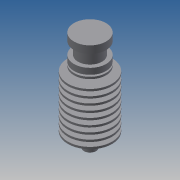
# Autodesk Inventor part: heat sink
Saved by Autodesk Inventor 2013 (Build 170138000, 138)
## iProperties
Created: 2017-04-01
Part Number: heat sink
Material: Generic
Document SubType Name: Modeling
Designer: employee
Density: 1 g/cm^3
Author: employee
Autodesk Inventor part; units mm, degrees
ref_plane "YZ Plane" through (0, 0, 0) normal (1, 0, 0) x (0, 1, 0)
ref_plane "XZ Plane" through (0, 0, 0) normal (0, 1, 0) x (-1, 0, 0)
ref_plane "XY Plane" through (0, 0, 0) normal (0, 0, 1) x (1, 0, 0)
sketch "Sketch1" plane through (0, 0, 0) normal (1, 0, 0) x (0, 1, 0)
  line L0 (0, -49.8) -> (0, 0)
  line L1 (0, 0) -> (-8, 0)
  line L2 (-8, 0) -> (-8, -3.7)
  line L3 (-8, -3.7) -> (-6, -3.7)
  line L4 (-6, -3.7) -> (-6, -9.7)
  line L5 (-6, -9.7) -> (-8, -9.7)
  line L6 (-8, -9.7) -> (-8, -12.7)
  line L7 (-8, -12.7) -> (-3, -12.7)
  line L8 (-3, -12.7) -> (-3, -49.8)
  line L9 (-3, -49.8) -> (0, -49.8)
  line L10 (-3, -42.7) -> (-11, -42.7)
  line L11 (-11, -42.7) -> (-11, -41.7)
  line L12 (-11, -41.7) -> (-3, -41.7)
  line L13 (-3, -41.7) -> (-3, -42.7)
  line L14 (-3, -39.575) -> (-11, -39.575)
  line L15 (-11, -39.575) -> (-11, -38.575)
  line L16 (-11, -38.575) -> (-3, -38.575)
  line L17 (-3, -38.575) -> (-3, -39.575)
  line L18 (-3, -27.075) -> (-11, -27.075)
  line L19 (-11, -27.075) -> (-11, -26.075)
  line L20 (-11, -26.075) -> (-3, -26.075)
  line L21 (-3, -26.075) -> (-3, -27.075)
  line L22 (-3, -20.825) -> (-11, -20.825)
  line L23 (-11, -20.825) -> (-11, -19.825)
  line L24 (-11, -19.825) -> (-3, -19.825)
  line L25 (-3, -19.825) -> (-3, -20.825)
  line L26 (-3, -30.2) -> (-11, -30.2)
  line L27 (-11, -30.2) -> (-11, -29.2)
  line L28 (-11, -29.2) -> (-3, -29.2)
  line L29 (-3, -29.2) -> (-3, -30.2)
  line L30 (-3, -33.325) -> (-11, -33.325)
  line L31 (-11, -33.325) -> (-11, -32.325)
  line L32 (-11, -32.325) -> (-3, -32.325)
  line L33 (-3, -32.325) -> (-3, -33.325)
  line L34 (-3, -36.45) -> (-11, -36.45)
  line L35 (-11, -36.45) -> (-11, -35.45)
  line L36 (-11, -35.45) -> (-3, -35.45)
  line L37 (-3, -35.45) -> (-3, -36.45)
  line L38 (-3, -23.95) -> (-11, -23.95)
  line L39 (-11, -23.95) -> (-11, -22.95)
  line L40 (-11, -22.95) -> (-3, -22.95)
  line L41 (-3, -22.95) -> (-3, -23.95)
  line L42 (-3, -17.7) -> (-11, -17.7)
  line L43 (-11, -17.7) -> (-11, -16.7)
  line L44 (-11, -16.7) -> (-3, -16.7)
  line L45 (-3, -16.7) -> (-3, -17.7)
  line L46 (-11, -17.7) -> (-11, -19.825) construction
  line L47 (-11, -20.825) -> (-11, -22.95) construction
  line L48 (-11, -23.95) -> (-11, -26.075) construction
  line L49 (-11, -27.075) -> (-11, -29.2) construction
  line L50 (-11, -30.2) -> (-11, -32.325) construction
  line L51 (-11, -33.325) -> (-11, -35.45) construction
  line L52 (-11, -36.45) -> (-11, -38.575) construction
  line L53 (-11, -41.7) -> (-11, -39.575) construction
  line L54 (-8, -13.575) -> (-3, -13.575)
  line L55 (-3, -13.575) -> (-3, -14.575)
  line L56 (-3, -14.575) -> (-8, -14.575)
  line L57 (-8, -14.575) -> (-8, -13.575)
  line L58 (-8, -14.575) -> (-8, -16.7) construction
  line L59 (-3, -42.7) -> (-2.05, -42.7)
  line L60 (-2.05, -42.7) -> (-2.05, -44.8)
  line L61 (-2.05, -44.8) -> (-3, -44.8)
  line L62 (-3, -44.8) -> (-3, -42.7)
  dimension "d0" = 3.7
  dimension "d2" = 6
  dimension "d3" = 3
  dimension "d4" = 8
  dimension "d5" = 6
  dimension "d6" = 3
  dimension "d7" = 49.8
  dimension "d9" = 1
  dimension "d11" = 26
  dimension "d12" = 7.1
  dimension "d13" = 11
  dimension "d14" = 5
  dimension "d15" = 2.05
  constraints: 124 end point, 30 parallel, 27 equal length, 12 perpendicular, 11 horizontal, 8 collinear, 2 vertical, 1 point on line, 13 other
  measures "d0" distance of L1.end L2.end
  measures "d2" distance of L3.end L4.end
  measures "d3" distance of L5.end L6.end
  measures "d4" distance of L0.end L1.end
  measures "d5" distance between parallel lines of L0 L4
  measures "d7" distance from line of L0.start L1
  measures "d9" distance of L10.end L11.end
  measures "d11" distance from line of L43.end L10
  measures "d12" distance between parallel lines of L10 L9
  measures "d13" distance from line of L10.end L0
  measures "d14" distance between parallel lines of L61 L9
  measures "d15" distance from line of L60.end L0
revolve "Revolution1" add sketch "Sketch1" angle 360 about axis through (0, 0, -49.8) along (0, 0, 1) contours L9 L8 L61 L60 L59 L7 L6 L5 L4 L3 L2 L1 L0 | L10 L11 L12 L8 | L14 L15 L16 L8 | L34 L35 L36 L8 | L8 L56 L57 L54 | L30 L31 L32 L8 | L8 L42 L43 L44 | L26 L27 L28 L8 | L8 L22 L23 L24 | L18 L19 L20 L8 | L8 L38 L39 L40
body "Solid1"
